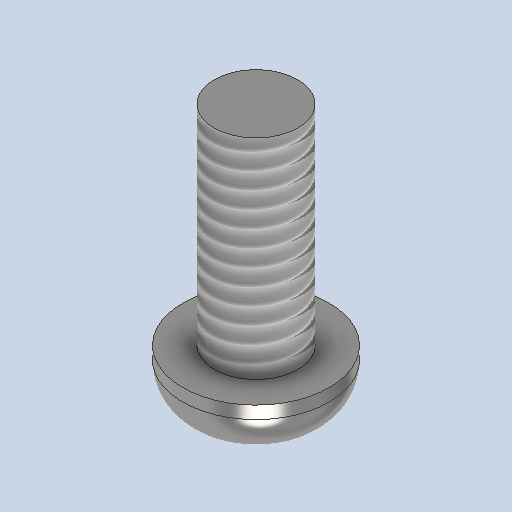
# Autodesk Inventor part: U-0205
Saved by Autodesk Inventor 2024.2 (Build 282272000, 272)
## iProperties
Part Number: U-0205
Material: Stainless Steel
Document SubType Name: Modeling
Designer: Masato Kubotera
Density: 8 g/cm^3
Appearance: Semi-Polished
Mass: 0.657 g
Surface Area: 1.94048 cm^2
Volume: 0.105552 cm^3
Vendor: NISSAN SCREW
Catalog Web Link: https://wilco.jp/products/U/U.html
Author: Masato Kubotera
Autodesk Inventor part; units mm, degrees
ref_plane "YZ Plane" through (0, 0, 0) normal (1, 0, 0) x (0, 1, 0)
ref_plane "XZ Plane" through (0, 0, 0) normal (0, 1, 0) x (-1, 0, 0)
ref_plane "XY Plane" through (0, 0, 0) normal (0, 0, 1) x (1, 0, 0)
sketch "スケッチ1" plane through (0, 0, 0) normal (1, 0, 0) x (0, 1, 0)
  line L0 (0, 6.3) -> (0, 0)
  line L1 (0, 0) -> (0.75, 0)
  line L2 (1.75, 1) -> (1.75, 1.3)
  line L3 (1.75, 1.3) -> (1, 1.3)
  line L4 (1, 1.3) -> (1, 6.3)
  line L5 (1, 6.3) -> (0, 6.3)
  line L6 (0.75, 0) -> (0, 1.3)
  arc A0 (0.75, 0) -> (1.75, 1) centre (0.75, 1) ccw
  line L7 (0.75, 0) -> (1.75, 0)
  line L8 (1.75, 0) -> (1.75, 1)
  dimension "d2" = 1.3
  dimension "d10" = 5
  dimension "d11" = 2
  dimension "d12" = 3.5
  dimension "d14" = 1
  constraints: 18 end point, 6 perpendicular, 4 point on line, 2 point on circle, 2 tangent, 1 centre point, 1 horizontal, 1 vertical
  measures "d2" distance of L7.end L2.end
  measures "d10" distance of L3.end L4.end
  measures "d11" diameter of L4 L0
  measures "d12" diameter of L2 L0
  measures "d14" radius of A0
revolve "回転1" add sketch "スケッチ1" angle 360 about axis through (0, 0, 6.3) along (0, 0, -1) contours L5 L4 L3 L2 A0 L6 L0
thread "ねじ1" size "M2x0.4" class "6g" standard "ANSI Metric M Profile" full length
sketch "スケッチ2" plane through (0, 0, 1.3) normal (0, 0, 1) x (1, 0, 0)
  line L0 (0.125, -1.7455) -> (-0.125, -1.7455)
  line L1 (-0.125, -1.7455) -> (-0.125, -0.375)
  line L2 (-0.125, 1.7455) -> (0.125, 1.7455)
  line L3 (0.125, 1.7455) -> (0.125, 0.375)
  line L4 (0.125, -1.7455) -> (-0.125, 1.7455) construction
  line L5 (-0.125, -1.7455) -> (0.125, 1.7455) construction
  line L6 (-1.7455, 0.125) -> (-0.375, 0.125)
  line L7 (1.7455, 0.125) -> (1.7455, -0.125)
  line L8 (1.7455, -0.125) -> (0.375, -0.125)
  line L9 (-1.7455, -0.125) -> (-1.7455, 0.125)
  line L10 (-1.7455, 0.125) -> (1.7455, -0.125) construction
  line L11 (1.7455, 0.125) -> (-1.7455, -0.125) construction
  line L12 (0.125, -0.375) -> (0.125, -1.7455)
  line L13 (0.375, 0.125) -> (1.7455, 0.125)
  line L14 (-0.375, -0.125) -> (-1.7455, -0.125)
  line L15 (-0.125, 0.375) -> (-0.125, 1.7455)
  arc A0 (0.375, -0.125) -> (0.125, -0.375) centre (0.375, -0.375) ccw
  arc A1 (0.125, 0.375) -> (0.375, 0.125) centre (0.375, 0.375) ccw
  arc A2 (-0.375, 0.125) -> (-0.125, 0.375) centre (-0.375, 0.375) ccw
  arc A3 (-0.125, -0.375) -> (-0.375, -0.125) centre (-0.375, -0.375) ccw
  circle A4 centre (0, 0) radius 1.75 projected
  line L16 (0, 1.75) -> (0, -1.75) construction
  line L17 (1.7455, 0) -> (-1.7455, 0) construction
  point P0 (-0.3339, -0.2226)
  point P1 (-0.3339, 0.2226)
  point P2 (0.3339, 0.2226)
  point P3 (0.3339, -0.2226)
  point P4 (0, 0)
  dimension "d18" = 0.25
  dimension "d19" = 0.25
  dimension "d20" = 0.25
  constraints: 36 end point, 12 point on circle, 10 parallel, 8 midpoint, 8 tangent, 4 centre point, 4 horizontal, 4 perpendicular, 3 equal radius, 1 vertical, 3 other
  measures "d18" radius of A0
  measures "d19" distance between parallel lines of L15 L3
  measures "d20" distance between parallel lines of L14 L6
extrude "押し出し2" add sketch "スケッチ2" against normal blind 1.3 contours A4 L0 | L12 A0 L8 A4 | A4 L14 A3 L1 | L7 A4 | A4 L9 | L13 A1 L3 A4 | A4 L15 A2 L6 | L2 A4
revolve "回転2" cut sketch "スケッチ1" angle 360 about axis through (0, 0, 6.3) along (0, 0, -1) contours A0 L8 L7
equation "\"d19\" = d20"
equation "\"d20\" = d18"
